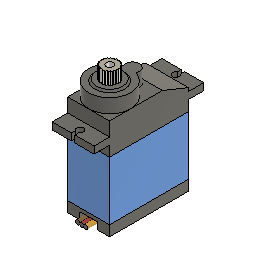
2307 MicroServo MG923B (Autodesk Fusion 360 design; units mm, degrees)
Autodesk Fusion 360 part; units mm, degrees
note: some values were not read from the file. Chosen so that the rebuilt part matches the saved one: which bodies a step acts on; which face or edge a step refers to. Set by a fixed rule: which sketch regions a step uses.
sketch "base" plane through (0, 0, 0) normal (0, 0, 1) x (1, 0, 0)
  circle A0 centre (0, 0) radius 2.25
  circle A1 centre (0, 0) radius 6
  line L0 (-6, 21) -> (6, 21)
  line L1 (6, 21) -> (6, -10.5)
  line L2 (6, -10.5) -> (-6, -10.5)
  line L3 (-6, -10.5) -> (-6, 21)
  line L4 (0, -10.5) -> (0, 0) construction
  line L5 (0, 0) -> (0, 6.5) construction
  circle A2 centre (0, 6.5) radius 2
  line L6 (-6, 16.55) -> (6, 16.55)
  line L7 (-6, -6.05) -> (6, -6.05)
  circle A3 centre (0, 19) radius 1
  line L8 (0, 19) -> (0, 21) construction
  line L9 (-0.5, 21) -> (-0.5, 19.866)
  line L10 (0.5, 21) -> (0.5, 19.866)
  line L11 (6, 5.25) -> (14, 5.25) construction
  line L12 (0.5, -10.5) -> (0.5, -9.366)
  line L13 (-0.5, -10.5) -> (-0.5, -9.366)
  circle A4 centre (0, -8.5) radius 1
  circle A5 centre (0, 0) radius 4.25
  dimension "d1" = 12
  dimension "d2" = 31.5
  dimension "d3" = 4.5
  dimension "d4" = 12
  dimension "d5" = 10.5
  dimension "d7" = 4
  dimension "d8" = 6.5
  dimension "d9" = 22.6
  dimension "d10" = 4.45
  dimension "d18" = 2
  dimension "d19" = 2
  dimension "d21" = 0.5
  dimension "d51" = 2
  constraint coincident A0.centre A1.centre
  constraint horizontal L0
  constraint vertical L1
  constraint horizontal L2
  constraint vertical L3
  constraint midpoint L2 L4.start
  constraint vertical L4
  constraint parallel L4 L5
  constraint coincident L5.end A2.centre
  constraint coincident L3 L6.start
  constraint perpendicular L3 L6
  constraint coincident L3 L7.start
  constraint coincident L1 L7.end
  constraint perpendicular L1 L7
  constraint coincident A3.centre L8.start
  constraint midpoint L0 L8.end
  constraint vertical L8
  constraint coincident L0 L9.start
  constraint perpendicular L0 L9
  constraint coincident A3 L9.end
  constraint symmetric L8 L9.start L10.start
  constraint symmetric L8 L9.end L10.end
  constraint midpoint L1 L11.start
  constraint perpendicular L1 L11
  constraint symmetric A3 L11 A4
  constraint symmetric L9.start L11 L13.start
  constraint symmetric L9.end L11 L13.end
  constraint symmetric L10.start L11 L12.start
  constraint symmetric L10.end L11 L12.end
  constraint concentric A0 A5
  measures "d1" distance of L0.start L0.end
  measures "d2" distance of L0.end L1.end
  measures "d3" diameter of A0
  measures "d4" diameter of A1
  measures "d5" distance of L4.start A0.centre
  measures "d7" diameter of A2
  measures "d8" distance of A0.centre L5.end
  measures "d9" distance of L6 L7
  measures "d10" distance of L0 L6
  measures "d18" diameter of A3
  measures "d19" distance of A3.centre L8.end
  measures "d21" distance of L8 L9
  measures "d51" distance of A0 A5
extrude "Extrude1" add sketch "base" against normal blind 22.8 contours A0 | A1 A2 | A1 L1 L3 L7 | A1 L1 L3 A2 L6 | A1 A2 | A1 A2 | A5 makes body 1 in component "body"
extrude "Extrude2" add sketch "base" along normal blind 2 contours A0 | A1 A2 | A1 L1 L3 L7 | A1 L1 L3 A2 L6 | A1 A2 | A1 A2 | L0 L1 L3 L6 A3 L9 L10 | L1 L2 L3 L7 L12 L13 A4 | A5 bodies 1 in component "body"
ref_plane "WorkPlane1" through (0, 5.25, -19.8) normal (0, 0, -1) x (-1, 0, 0) in component "body"
ref_plane "WorkPlane2" through (0, 5.25, -3) normal (0, 0, 1) x (1, 0, 0) in component "body"
split "Split1" by plane through (0, 5.25, -3) normal (0, 0, 1) and through (0, 5.25, -19.8) normal (0, 0, -1) bodies 1 makes body 2 at (2, 9.0167, -22.8) makes body 3 at (-4.2078, 0.9273, 2) in component "body"
sketch "Sketch1" plane through (0, 0, 0) normal (1, 0, 0) x (0, 1, 0) in component "body"
  line L0 (16.55, 2) -> (16.55, 3)
  line L1 (16.55, 3) -> (9.1247, 6)
  line L2 (9.1247, 6) -> (-6.05, 6)
  line L3 (-6.05, 6) -> (-6.05, 2)
  line L4 (-6.05, 2) -> (16.55, 2)
  line L5 (-6.05, 0) -> (-6.05, -3)
  line L6 (16.55, 0) -> (16.55, -3)
  dimension "d40" = 1
  dimension "d41" = 112
  dimension "d44" = 2
  dimension "d45" = 4
  constraint vertical L0
  constraint perpendicular L0 L2
  constraint perpendicular L2 L3
  constraint collinear L3 L5
  constraint collinear L0 L6
  constraint horizontal L4
  measures "d40" distance of L0.start L0.end
  measures "d41" angle of L0 L1
  measures "d44" distance of origin L4
  measures "d45" distance of L2.end L3.end
extrude "Extrude3" add sketch "Sketch1" along normal mid plane 12 bodies 3 in component "body"
extrude "Extrude4" add sketch "base" along normal blind 4 from surface at 6 contours A0 | A1 A2 | A1 A2 | A1 A2 | A5 bodies 3 in component "body"
extrude "Extrude5" add sketch "base" along normal blind 0.5 draft -45 from surface at 10 contours A0 | A5 bodies 3 in component "body"
extrude "Extrude6" cut sketch "base" against normal blind 4.5 from surface at 10.5 contours A0 bodies 3 in component "body"
ref_plane "WorkPlane1" through (0, 0, 6) normal (0, 0, 1) x (1, 0, 0) in component "spline"
sketch "spline" plane through (0, 0, 6) normal (0, 0, 1) x (1, 0, 0)
  circle A0 centre (0, 0) radius 2.2
  line L0 (2.5, 0) -> (2, 0.5)
  line L1 (2, 0.5) -> (2, -0.5)
  line L2 (2, -0.5) -> (2.5, 0)
  line L3 (2.5, 0) -> (2, 0) construction
  line L4 (2, 0) -> (0, 0) construction
  circle A1 centre (0, 0) radius 1
  dimension "d59" = 4.4
  dimension "d62" = 45
  dimension "d63" = 0.5
  dimension "d64" = 2
  dimension "d75" = 2
  constraint coincident A0.centre L4.end
  constraint vertical L1
  constraint perpendicular L0 L2
  constraint midpoint L1 L3.end
  constraint perpendicular L1 L3
  constraint horizontal L4
  constraint concentric A0 A1
  measures "d59" diameter of A0
  measures "d62" angle of L0 L1
  measures "d63" distance of L0.start L3.end
  measures "d64" distance of L3.end A0.centre
  measures "d75" diameter of A1
extrude "Extrude1'" add sketch "spline" along normal blind 4.5 separate body contours A0 L0 L1 L2 | A0 L0 L1 L2 | A1 makes body 4 in component "spline"
extrude "Extrude2'" add sketch "spline" along normal blind 3.5 from surface at 4.5 separate body contours A0 L0 L1 L2 | A0 L0 L1 L2 makes body 5 in component "spline"
extrude "Extrude3'" add sketch "spline" along normal up to surface (3.5 mm away) from surface at 4.5 contours A0 L0 L2 bodies 5 in component "spline"
pattern_circular "C-Pattern1" count 22 over 360 about axis through (0, 0, 10.5) along (0, 0, 1) of "Extrude3'" in component "spline"
sketch "Sketch2" plane through (0, 0, -22.8) normal (0, 0, -1) x (1, 0, 0) in component "body"
  line L0 (6, 6.05) -> (-6, 6.05)
  line L1 (2.5, 6.05) -> (-2.5, 6.05)
  line L2 (-2.5, 6.05) -> (-2.5, 4.05)
  line L3 (-2.5, 4.05) -> (2.5, 4.05)
  line L4 (2.5, 4.05) -> (2.5, 6.05)
  dimension "d88" = 5
  dimension "d89" = 2
  constraint horizontal L1
  constraint vertical L2
  constraint horizontal L3
  constraint vertical L4
  constraint midpoint L0 L1
  measures "d88" distance of L2.end L3.end
  measures "d89" distance of L1.start L3.end
extrude "Extrude8" cut sketch "Sketch2" against normal blind 2 bodies 2 in component "body"
sketch "Sketch3" plane through (0, -4.05, 0) normal (0, -1, 0) x (1, 0, 0) in component "body"
  line L0 (-2.5, -22.8) -> (-2.5, -20.8)
  line L1 (2.5, -22.8) -> (2.5, -20.8)
  line L2 (2.5, -21.8) -> (-2.5, -21.8) construction
  circle A0 centre (0, -21.8) radius 0.6
  circle A1 centre (1.1, -21.8) radius 0.6
  circle A2 centre (-1.1, -21.8) radius 0.6
  dimension "d92" = 1.2
  dimension "d93" = 1.2
  dimension "d94" = 1.1
  dimension "d95" = 1.2
  dimension "d96" = 1.1
  constraint midpoint L1 L2.start
  constraint midpoint L0 L2.end
  constraint midpoint L2 A0.centre
  constraint coincident L2 A1.centre
  constraint coincident L2 A2.centre
  measures "d92" diameter of A0
  measures "d93" diameter of A1
  measures "d94" distance of A0.centre A1.centre
  measures "d95" diameter of A2
  measures "d96" distance of A0.centre A2.centre
extrude "Extrude9" add sketch "Sketch3" along normal blind 4 separate body makes body 6 in component "body"
component "body" placed x (1, 0, 0) y (0, 1, 0) z (0, 0, 1) at (0, 0, 0)
component "spline" placed x (1, 0, 0) y (0, 1, 0) z (0, 0, 1) at (0, 0, 0)
